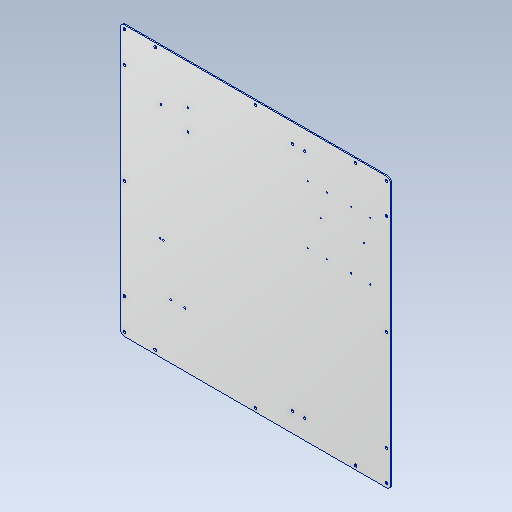
# Autodesk Inventor part: 0008-10-022 Tabla suport
Saved by Autodesk Inventor 2020 (Build 240168000, 168)
## iProperties
Created: 2021-03-06
Part Number: 0008-10-022 Tabla suport
Material: Aluminum 6061
Document SubType Name: Modeling
Designer: Iulian Bors
Density: 2.7 g/cm^3
Appearance: Aluminum - Flat
Mass: 3961.63 g
Surface Area: 9881.05 cm^2
Volume: 1467.27 cm^3
Description: Placa rigidizare
Author: Iulian Bors
Subject: 022
Autodesk Inventor part; units mm, degrees
ref_plane "YZ Plane" through (0, 0, 0) normal (1, 0, 0) x (0, 1, 0)
ref_plane "XZ Plane" through (0, 0, 0) normal (0, 1, 0) x (-1, 0, 0)
ref_plane "XY Plane" through (0, 0, 0) normal (0, 0, 1) x (1, 0, 0)
sketch "Sketch1" plane through (0, 0, 0) normal (0, 0, 1) x (1, 0, 0)
  line L0 (-350, 350) -> (350, 350)
  line L1 (350, 350) -> (350, -350)
  line L2 (350, -350) -> (-350, -350)
  line L3 (-350, -350) -> (-350, 350)
  point P0 (0, 0)
  point P1 (0, 350)
  point P2 (-350, 0)
  dimension "d0" = 700
  dimension "d1" = 700
  constraints: 8 end point, 2 midpoint, 2 parallel, 1 horizontal, 1 horizontal alignment, 1 perpendicular, 1 vertical alignment
  measures "d0" distance of L0.start L0.end
  measures "d1" distance of L2.end L0.start
extrude "Extrusion1" add sketch "Sketch1" along normal blind 3
sketch "Sketch2" plane through (0, 0, 3) normal (0, 0, 1) x (1, 0, 0)
  line L0 (-340, 340) -> (340, 340) construction
  line L1 (340, 340) -> (340, -340) construction
  line L2 (340, -340) -> (-340, -340) construction
  line L3 (-340, -340) -> (-340, 340) construction
  line L4 (350, 350) -> (-350, 350) construction
  line L5 (350, -350) -> (350, 350) construction
  point P0 (0, 0)
  point P1 (0, 340)
  point P2 (340, 0)
  point P3 (-340, 260)
  point P4 (-340, -260)
  point P5 (-260, -340)
  point P6 (260, -340)
  point P7 (340, -260)
  point P8 (340, 260)
  point P9 (260, 340)
  point P10 (-260, 340)
  point P11 (-340, 0)
  point P12 (340, 0)
  point P13 (0, 340)
  point P14 (0, -340)
  dimension "d4" = 10
  dimension "d5" = 10
  dimension "d6" = 340
  dimension "d8" = 80
  dimension "d10" = 80
  dimension "d11" = 80
  dimension "d12" = 80
  dimension "d13" = 80
  dimension "d14" = 80
  dimension "d15" = 80
  dimension "d16" = 80
  constraints: 8 end point, 8 point on line, 5 midpoint, 2 horizontal alignment, 2 parallel, 1 coincident, 1 horizontal, 1 perpendicular, 1 vertical alignment
  measures "d4" distance between parallel lines of L4 L0
  measures "d5" distance between parallel lines of L5 L1
  measures "d6" distance from line of point (0, 0) L0
  measures "d8" distance of L0.start point (-340, 260)
  measures "d10" distance of L0.start point (-260, 340)
  measures "d11" distance of L2.end point (-340, -260)
  measures "d12" distance of point (-260, -340) L2.end
  measures "d13" distance of L1.end point (260, -340)
  measures "d14" distance of L1.end point (340, -260)
  measures "d15" distance of point (340, 260) L0.end
  measures "d16" distance from line of L1 point (260, 340)
hole "Hole1" at (-340, 340, 3) at (340, -340, 3) at (340, 340, 3) at (-340, -340, 3) at (-340, 260, 3) at (-340, -260, 3) at (-260, -340, 3) at (260, -340, 3) at (340, -260, 3) at (340, 260, 3) at (260, 340, 3) at (-260, 340, 3) at (-340, 0, 3) at (340, 0, 3) at (0, -340, 3) at (0, 340, 3) direction (0, 0, -1) diameter 7 end through all
sketch "Sketch3" plane through (0, 0, 3) normal (0, 0, 1) x (1, 0, 0)
  circle A0 centre (127.972, -300) radius 3.4 projected
  circle A1 centre (95.972, -300) radius 3.4 projected
  circle A2 centre (127.972, 300) radius 3.4 projected
  circle A3 centre (95.972, 300) radius 3.4 projected
  circle A4 centre (298.5, 236) radius 1.5
  circle A5 centre (248.5, 236) radius 1.5
  circle A6 centre (282, 171) radius 1.5
  circle A7 centre (248.5, 86) radius 1.5
  line L0 (317, 136) -> (296, 136) projected
  circle A8 centre (298.5, 86) radius 1.5
  circle A9 centre (135.5, 236) radius 1.5
  circle A10 centre (185.5, 236) radius 1.5
  circle A11 centre (169, 171) radius 1.5
  circle A12 centre (135.5, 86) radius 1.5
  line L1 (182, 93.5) -> (189.5, 93.5) projected
  circle A13 centre (185.5, 86) radius 1.5
  circle A14 centre (-175, 276.5) radius 2 projected
  circle A15 centre (-175, 161.5) radius 2 projected
  circle A16 centre (-245, 161.5) radius 2 projected
  circle A17 centre (-245, 276.5) radius 2 projected
  circle A18 centre (-220, -208) radius 2.5 projected
  circle A19 centre (-183, -208) radius 2.5 projected
  line L2 (-250, -88.5) -> (-250, -77.5) projected
  line L3 (-240, -88.5) -> (-250, -88.5) projected
  line L4 (-250, -77.5) -> (-240, -77.5) projected
  circle A20 centre (-247, -83) radius 2
  circle A21 centre (-239, -83) radius 2
  line L5 (-250, 171.5) -> (-250, 266.5) projected
  circle A22 centre (-245, 219) radius 2.5 projected
  circle A23 centre (-175, 246.5) radius 2.5 projected
  circle A24 centre (-175, 191.5) radius 2.5 projected
  line L6 (248.5, 86) -> (298.5, 86)
  line L7 (298.5, 86) -> (298.5, 236)
  line L8 (298.5, 236) -> (248.5, 236)
  line L9 (248.5, 236) -> (248.5, 86)
  line L10 (350, 350) -> (-350, 350) projected
  line L11 (350, -350) -> (350, 350) projected
  line L12 (135.5, 86) -> (185.5, 86)
  line L13 (185.5, 86) -> (185.5, 236)
  line L14 (185.5, 236) -> (135.5, 236)
  line L15 (135.5, 236) -> (135.5, 86)
  point P0 (0, 0)
  point P1 (200.5, 93.5)
  point P2 (191, 93.5)
  point P3 (-250, -83)
  dimension "d27" = 4
  dimension "d28" = 4
  dimension "d29" = 8
  dimension "d30" = 3
  dimension "d31" = 3
  dimension "d32" = 16.5
  dimension "d33" = 65
  dimension "d34" = 114
  dimension "d35" = 150
  dimension "d36" = 51.5
  dimension "d37" = 50
  dimension "d38" = 16.5
  dimension "d39" = 65
  dimension "d40" = 63
  dimension "d41" = 114
  dimension "d42" = 150
  dimension "d43" = 50
  constraints: 16 end point, 12 centre point, 9 equal radius, 4 coincident, 4 parallel, 2 horizontal, 2 horizontal alignment, 2 perpendicular, 1 midpoint, 2 other
  measures "d27" diameter of A20
  measures "d28" diameter of A21
  measures "d29" distance of A20.centre A21.centre
  measures "d30" distance from line of L2 A20.centre
  measures "d31" diameter of A7
  measures "d32" distance from line of L7 A6.centre
  measures "d33" distance from line of L8 A6.centre
  measures "d34" distance between parallel lines of L10 L8
  measures "d35" distance of L8.end L6.start
  measures "d36" distance between parallel lines of L11 L7
  measures "d37" distance of L6.start L6.end
  measures "d38" distance from line of L13 A11.centre
  measures "d39" distance from line of L14 A11.centre
  measures "d40" distance between parallel lines of L9 L13
  measures "d41" distance between parallel lines of L10 L14
  measures "d42" distance of L12.end L13.end
  measures "d43" distance of L12.start L12.end
extrude "Extrusion2" cut sketch "Sketch3" against normal through all contours A0 | A1 | A2 | A3 | A4 L7 L8 | L8 L7 A4 | L8 L9 A5 | A5 L9 L8 | L7 L6 A8 | A8 L6 L7 | L9 L6 A7 | A7 L6 L9 | A6 | L14 L15 A9 | A9 L15 L14 | L14 L13 A10 | A10 L13 L14 | L15 L12 A12 | A12 L12 L15 | L12 L13 A13 | A13 L13 L12 | A11 | A18 | A19 | A20 | A21 | A22 | A23 | A24
fillet "Fillet1" radius 10 4 edges at (-350, -350, 1.5) (-350, 350, 1.5) (350, 350, 1.5) (350, -350, 1.5)
equation "\"d10\" = d8"
equation "\"d11\" = d8"
equation "\"d12\" = d8"
equation "\"d13\" = d8"
equation "\"d14\" = d8"
equation "\"d15\" = d8"
equation "\"d16\" = d8"
equation "\"d7\" = 0.333333 * d6"
body "Solid1"
